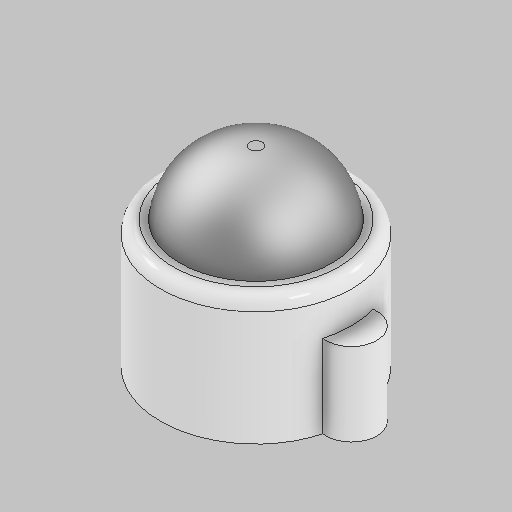
# Autodesk Inventor part: Rueda Loca
Saved by Autodesk Inventor 2025 (Build 290162010, 162A)
## iProperties
Created: 2024-06-08
Part Number: Rueda Loca
Material: Genérico
Document SubType Name: Sheet Metal
Designer: juesr
Density: 1 g/cm^3
Sheet Metal Rule: Por defecto_mm
Appearance: Valor por defecto
Author: juesr
Autodesk Inventor part; units mm, degrees
ref_plane "YZ Plane" through (0, 0, 0) normal (1, 0, 0) x (0, 1, 0)
ref_plane "XZ Plane" through (0, 0, 0) normal (0, 1, 0) x (-1, 0, 0)
ref_plane "XY Plane" through (0, 0, 0) normal (0, 0, 1) x (1, 0, 0)
sketch "Boceto1" plane through (0, 0, 0) normal (0, 1, 0) x (-1, 0, 0)
  circle A0 centre (0, 0) radius 6
  dimension "d0" = 0
  dimension "d1" = 0
  dimension "d2" = 12
  constraints: 1 centre point
  measures "d0" distance of point (0, 0) A0.centre
  measures "d1" distance of A0.centre point (0, 0)
  measures "d2" diameter of A0
extrude "Extrusión1" add sketch "Boceto1" along normal blind 15
fillet "Empalme1" radius 5.5 1 edges at (6, 15, 0)
sketch "Boceto2" plane through (0, 0, 0) normal (0, -1, 0) x (1, 0, 0)
  circle A0 centre (0, 0) radius 7.5
  dimension "d6" = 15
  constraints: 1 centre point, 1 coincident
  measures "d6" diameter of A0
extrude "Extrusión2" add sketch "Boceto2" against normal blind 10
fillet "Empalme2" radius 1 1 edges at (-7.5, 10, 0)
sketch "Boceto3" plane through (0, 0, 0) normal (0, -1, 0) x (1, 0, 0)
  circle A0 centre (0, 0) radius 6.5 projected
  circle A1 centre (7.5, 0) radius 2
  circle A2 centre (-7.5, 0) radius 2
  dimension "d10" = 7.5
  dimension "d12" = 4
  dimension "d14" = 7.5
  dimension "d15" = 4
  constraints: 2 centre point
  measures "d10" distance of point (0, 0) A1.centre
  measures "d12" diameter of A1
  measures "d14" distance of A2.centre point (0, 0)
  measures "d15" diameter of A2
extrude "Extrusión3" add sketch "Boceto3" against normal blind 6.5 contours A0 A1 | A0 A1 | A2 A0 | A0 A2
equation "\"Radio_pliegue\" = Grosor"
equation "\"Anchura_desahogo_plegado\" = Grosor"
equation "\"Profundidad_desahogo_plegado\" = 0.5 * Grosor"
equation "\"Tamaño_destalonado\" = 4 * Grosor"
equation "\"Remanente_mínimo\" = 2 * Grosor"
equation "\"Radiodetransición\" = Radio_pliegue"
equation "\"Tamaño_de_radio_de_Jacobi\" = Radio_pliegue"
equation "\"TamañoSeparación\" = Grosor"
equation "\"Grosor\" = 0.5"
